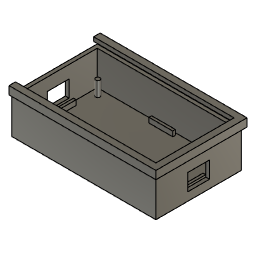
KrabickaSpodek (Autodesk Fusion 360 design; units mm, degrees)
Autodesk Fusion 360 part; units mm, degrees
sketch "Spodek" plane through (0, 0, 0) normal (0, 0, 1) x (1, 0, 0)
  line L0 (0, 0) -> (61, 0)
  line L1 (61, 0) -> (61, 34)
  line L2 (61, 34) -> (0, 34)
  line L3 (0, 34) -> (0, 0)
  line L4 (-1, 35) -> (62, 35)
  line L5 (62, 35) -> (62, -1)
  line L6 (62, -1) -> (-1, -1)
  line L7 (-1, -1) -> (-1, 35)
  line L8 (-2.7, -2.7) -> (-2.7, 36.7) construction
  line L9 (63.7, 36.7) -> (-2.7, 36.7) construction
  line L10 (63.7, -2.7) -> (63.7, 36.7) construction
  line L11 (63.7, -2.7) -> (-2.7, -2.7) construction
  line L12 (-2.7, -2.7) -> (63.7, -2.7)
  line L13 (63.7, -2.7) -> (63.7, 36.7)
  line L14 (63.7, 36.7) -> (-2.7, 36.7)
  line L15 (-2.7, 36.7) -> (-2.7, -2.7)
  dimension "d1" = 61
  dimension "d2" = 34
  dimension "d3" = 63
  dimension "d4" = 36
  dimension "d5" = 1.7
  dimension "d6" = 1.7
  dimension "d7" = 1.7
  dimension "d8" = 1.7
  constraint horizontal L0
  constraint vertical L1
  constraint horizontal L2
  constraint vertical L3
  constraint coincident L0.start L3.end
  constraint horizontal L4
  constraint vertical L5
  constraint horizontal L6
  constraint vertical L7
  constraint vertical L8
  constraint perpendicular L8 L9
  constraint perpendicular L9 L10
  constraint perpendicular L10 L11
  constraint horizontal L12
  constraint vertical L13
  constraint horizontal L14
  constraint vertical L15
  measures "d1" distance of L0.start L0.end
  measures "d2" distance of L0.start L2.end
  measures "d3" distance of L4.start L4.end
  measures "d4" distance of L4.start L6.end
  measures "d5" distance of L7 L8
  measures "d6" distance of L4 L9
  measures "d7" distance of L5 L10
  measures "d8" distance of L6 L11
sketch "TotoNevim" plane through (0, 0, 0) normal (0, 0, 1) x (1, 0, 0)
extrude "Extrude1" add sketch "Spodek" along normal blind 12 contours L12 L13 L14 L15 makes body 1
extrude "Extrude2" add sketch "Spodek" along normal blind 1.5 contours L0 L1 L2 L3 | L4 L5 L6 L7 bodies 1
sketch "Sketch3" plane through (0, 0, 1.5) normal (0, 0, 1) x (-1, 0, 0)
  line L0 (1, 1) -> (-62, 1)
  line L1 (-62, 1) -> (-62, -35)
  line L2 (-62, -35) -> (1, -35)
  line L3 (1, -35) -> (1, 1)
  line L4 (-59.78, -32.78) -> (-1.22, -32.78)
  line L5 (-1.22, -32.78) -> (-1.22, -1.22)
  line L6 (-1.22, -1.22) -> (-59.78, -1.22)
  line L7 (-59.78, -1.22) -> (-59.78, -32.78)
  line L8 (-61, 0) -> (-61, -34)
  line L9 (0, 0) -> (-61, 0)
  line L10 (0, -34) -> (0, 0)
  line L11 (-61, -34) -> (0, -34)
  dimension "d13" = 1.22
  dimension "d14" = 1.22
  dimension "d15" = 1.22
  dimension "d16" = 1.22
  constraint horizontal L4
  constraint vertical L5
  constraint horizontal L6
  constraint vertical L7
  measures "d13" distance of L7 L8
  measures "d14" distance of L6 L9
  measures "d15" distance of L5 L10
  measures "d16" distance of L4 L11
extrude "Extrude3" add sketch "Sketch3" along normal blind 1.8 contours L8 L9 L10 L11 bodies 1
extrude "Extrude4" add 1 faces at (20, -2.1333, 12) along direction (0, 0, 1) blind 5.243 on bodies 1 bodies 1
extrude "Extrude5" add 1 faces at (20, -2.1333, 17.243) along direction (0, 0, 1) blind 0.021 on bodies 1 bodies 1
sketch "Prurez1" plane through (-2.7, 0, 0) normal (-1, 0, 0) x (0, -1, 0)
  line L0 (-36.7, 0) -> (2.7, 0)
  line L1 (2.7, 0) -> (2.7, 17.264)
  line L2 (2.7, 17.264) -> (-36.7, 17.264)
  line L3 (-36.7, 17.264) -> (-36.7, 0)
  line L4 (-12, 3.3) -> (-12, 11) construction
  line L5 (0, 1.5) -> (0, 3.3) construction
  line L6 (-22, 11) -> (-22, 3.3) construction
  line L7 (-34, 3.3) -> (-34, 11) construction
  line L8 (-35, 1.5) -> (-35, 17.264) construction
  line L9 (-22, 11) -> (-12, 11) construction
  line L10 (-12, 11) -> (-12, 3.3) construction
  line L11 (-12, 3.3) -> (-22, 3.3) construction
  line L12 (-22, 3.3) -> (-22, 11) construction
  line L13 (-22, 11) -> (-12, 11)
  line L14 (-12, 11) -> (-12, 3.3)
  line L15 (-12, 3.3) -> (-22, 3.3)
  line L16 (-22, 3.3) -> (-22, 11)
  dimension "d23" = 7.7
  dimension "d24" = 12
  dimension "d25" = 12
  dimension "d26" = 1
  constraint perpendicular L2 L4
  constraint parallel L4 L6
  constraint perpendicular L2 L7
  constraint horizontal L9
  constraint vertical L10
  constraint horizontal L11
  constraint vertical L12
  constraint horizontal L13
  constraint vertical L14
  constraint horizontal L15
  constraint vertical L16
  measures "d23" distance of L4.start L4.end
  measures "d24" distance of L4 L5
  measures "d25" distance of L6 L7
  measures "d26" distance of L7 L8
extrude "Extrude6" cut sketch "Prurez1" against normal up to surface (66.4 mm away) contours L13 L14 L15 L16 bodies 1
sketch "Sketch5" plane through (0, 0, 17.264) normal (0, 0, 1) x (-1, 0, 0)
  line L0 (-62, 1) -> (1, 1)
  line L1 (1, 1) -> (1, -35)
  line L2 (1, -35) -> (-62, -35)
  line L3 (-62, -35) -> (-62, 1)
  line L4 (2.7, -36.7) -> (2.7, 2.7)
  line L5 (2.7, 2.7) -> (-63.7, 2.7)
  line L6 (-63.7, 2.7) -> (-63.7, -36.7)
  line L7 (-63.7, -36.7) -> (2.7, -36.7)
  line L8 (2.7, -36.7) -> (-63.7, -36.7)
  line L9 (-63.7, -36.7) -> (-63.7, 2.7)
  line L10 (-63.7, 2.7) -> (2.7, 2.7)
  line L11 (2.7, 2.7) -> (2.7, -36.7)
  line L12 (1, -35) -> (-62, -35)
  line L13 (-62, -35) -> (-62, 1)
  line L14 (-62, 1) -> (1, 1)
  line L15 (1, 1) -> (1, -35)
  constraint horizontal L8
  constraint vertical L9
  constraint horizontal L10
  constraint vertical L11
  constraint coincident L5.end L6.start
  constraint coincident L4.start L7.end
  constraint horizontal L12
  constraint vertical L13
  constraint horizontal L14
  constraint vertical L15
  constraint coincident L0.start L3.end
  constraint coincident L1.end L2.start
extrude "Extrude7" add sketch "Sketch5" along normal blind 3.7 bodies 1
sketch "Sketch6" plane through (-2.7, 0, 0) normal (-1, 0, 0) x (0, -1, 0)
  line L0 (-22, 3.3) -> (-22, 11)
  line L1 (-22, 11) -> (-12, 11)
  line L2 (-12, 11) -> (-12, 3.3)
  line L3 (-12, 3.3) -> (-22, 3.3)
  line L4 (-36.7, 0) -> (2.7, 0)
  line L5 (2.7, 0) -> (2.7, 20.964)
  line L6 (2.7, 20.964) -> (-36.7, 20.964)
  line L7 (-36.7, 20.964) -> (-36.7, 0)
  line L8 (-35, 17.264) -> (1.0001, 17.264)
  line L9 (1.0001, 17.264) -> (1.0001, 20.964)
  line L10 (1.0001, 20.964) -> (-35, 20.964)
  line L11 (-35, 20.964) -> (-35, 17.264)
  line L12 (-36.7, 17.264) -> (2.7, 17.264)
  constraint horizontal L8
  constraint vertical L9
  constraint horizontal L10
  constraint vertical L11
  constraint coincident L6 L9.end
  constraint coincident L8.start L12
extrude "Extrude8" cut sketch "Sketch6" against normal up to surface (64.7 mm away) contours L6 L8 L9 L10 L11 L12 bodies 1
sketch "BokFront" plane through (0, -2.7, 0) normal (0, -1, 0) x (1, 0, 0)
  line L0 (-2.7, 0) -> (63.7, 0)
  line L1 (63.7, 0) -> (63.7, 20.964)
  line L2 (63.7, 20.964) -> (-2.7, 20.964)
  line L3 (-2.7, 20.964) -> (-2.7, 0)
  line L4 (-2.7, 20.964) -> (63.7, 20.964)
  line L5 (63.7, 20.964) -> (63.7, 17.264)
  line L6 (63.7, 17.264) -> (-2.7, 17.264)
  line L7 (-2.7, 17.264) -> (-2.7, 20.964)
  point P0 (63.7, 17.264)
  constraint horizontal L4
  constraint vertical L5
  constraint horizontal L6
  constraint vertical L7
  constraint coincident P0 L5.end
  constraint coincident L2.end L3.start
sketch "BokRight" plane through (63.7, 0, 0) normal (1, 0, 0) x (0, 1, 0)
  line L0 (22, 11) -> (22, 3.3)
  line L1 (22, 3.3) -> (12, 3.3)
  line L2 (12, 3.3) -> (12, 11)
  line L3 (12, 11) -> (22, 11)
  line L4 (-2.7, 0) -> (36.7, 0)
  line L5 (36.7, 0) -> (36.7, 20.964)
  line L6 (36.7, 20.964) -> (-2.7, 20.964)
  line L7 (-2.7, 20.964) -> (-2.7, 0)
  line L8 (-2.7, 20.964) -> (36.7, 20.964)
  line L9 (36.7, 20.964) -> (36.7, 17.264)
  line L10 (36.7, 17.264) -> (-2.7, 17.264)
  line L11 (-2.7, 17.264) -> (-2.7, 20.964)
  point P0 (36.7, 17.264)
  constraint horizontal L8
  constraint vertical L9
  constraint horizontal L10
  constraint vertical L11
  constraint coincident P0 L9.end
  constraint coincident L6.end L7.start
sketch "BokBack" plane through (0, 36.7, 0) normal (0, 1, 0) x (-1, 0, 0)
  line L0 (-63.7, 0) -> (2.7, 0)
  line L1 (2.7, 0) -> (2.7, 20.964)
  line L2 (2.7, 20.964) -> (-63.7, 20.964)
  line L3 (-63.7, 20.964) -> (-63.7, 0)
  line L4 (-63.7, 20.964) -> (2.7, 20.964)
  line L5 (2.7, 20.964) -> (2.7, 17.264)
  line L6 (2.7, 17.264) -> (-63.7, 17.264)
  line L7 (-63.7, 17.264) -> (-63.7, 20.964)
  point P0 (2.7, 17.264)
  constraint horizontal L4
  constraint vertical L5
  constraint horizontal L6
  constraint vertical L7
  constraint coincident P0 L5.end
  constraint coincident L2.end L3.start
extrude "Extrude9" add sketch "BokBack" along normal blind 1.3 contours L1 L2 L3 L4 L5 L6 L7 bodies 1
extrude "Extrude10" add sketch "BokFront" along normal blind 1.3 contours L1 L2 L3 L4 L5 L6 L7 bodies 1
extrude "Extrude11" add sketch "BokRight" along normal blind 1.3 contours L5 L6 L7 L8 L9 L10 L11 bodies 1
extrude "Extrude12" add 1 faces at (63.7, 37.5667, 19.7307) along direction (1, 0, 0) blind 1.3 on bodies 1 bodies 1
extrude "Extrude13" add 1 faces at (63.7, -3.1333, 19.7307) along direction (1, 0, 0) blind 1.3 on bodies 1 bodies 1
sketch "Sketch10" plane through (-2.7, 0, 0) normal (-1, 0, 0) x (0, -1, 0)
  line L0 (-35, 17.264) -> (-35, 20.964)
  line L1 (-35, 20.964) -> (-38, 20.964)
  line L2 (-38, 20.964) -> (-38, 17.264)
  line L3 (-38, 17.264) -> (-36.7, 17.264)
  line L4 (-36.7, 17.264) -> (-36.7, 0)
  line L5 (-36.7, 0) -> (2.7, 0)
  line L6 (2.7, 0) -> (2.7, 17.264)
  line L7 (2.7, 17.264) -> (4, 17.264)
  line L8 (4, 17.264) -> (4, 20.964)
  line L9 (4, 20.964) -> (1.0001, 20.964)
  line L10 (1.0001, 20.964) -> (1.0001, 17.264)
  line L11 (1.0001, 17.264) -> (-35, 17.264)
  line L12 (-22, 3.3) -> (-22, 11)
  line L13 (-22, 11) -> (-12, 11)
  line L14 (-12, 11) -> (-12, 3.3)
  line L15 (-12, 3.3) -> (-22, 3.3)
  line L16 (4, 17.264) -> (2.7, 16)
  line L17 (-38, 17.264) -> (-36.7, 16)
  constraint coincident L7.end L8.start
  constraint coincident L6 L16.end
  constraint coincident L2.end L3.start
  constraint coincident L4 L17.end
extrude "Extrude14" add sketch "Sketch10" against normal up to surface (67.7 mm away) contours L3 L4 L17 | L6 L7 L16 bodies 1
sketch "Sketch11" plane through (0, -2.7, 0) normal (0, 1, 0) x (-1, 0, 0)
  line L0 (-63.7, 16) -> (-63.7, 17.264)
  line L1 (-63.7, 17.264) -> (-65, 17.264)
  line L2 (-65, 17.264) -> (-65, 16)
  line L3 (-65, 16) -> (-63.7, 16)
  line L4 (-65, 17.264) -> (-63.7, 16)
  constraint coincident L1.end L2.start
  constraint coincident L0.start L3.end
extrude "Extrude15" add sketch "Sketch11" along normal blind 39.4 contours L0 L1 L4 bodies 1
extrude "Extrude16" cut 1 faces at (64.5667, -2.7, 16.4213) along direction (0, -1, 0) blind 5.3 on bodies 1 bodies 1
extrude "Extrude17" cut 1 faces at (64.5667, 36.7, 16.4213) along direction (0, 1, 0) blind 1.9 on bodies 1 bodies 1
sketch "Sketch12" plane through (-2.7, 35.85, 19.114) normal (-1, 0, 0) x (0, -1, 0)
  line L0 (-0.85, 0) -> (0.85, 0)
  line L1 (0.85, 0) -> (0.85, -1.85)
  line L2 (0.85, -1.85) -> (-0.85, -1.85)
  line L3 (-0.85, -1.85) -> (-0.85, 0)
  line L4 (-0.85, 1.85) -> (-0.85, -19.114)
  line L5 (36.8501, -1.85) -> (38.55, -1.85)
  line L6 (38.55, -1.85) -> (38.55, 0)
  line L7 (38.55, 0) -> (36.8501, 0)
  line L8 (36.8501, 0) -> (36.8501, -1.85)
  line L9 (38.55, -19.114) -> (38.55, 1.85)
  point P0 (0.85, -1.85)
  point P1 (36.8501, -1.85)
  constraint horizontal L0
  constraint vertical L1
  constraint horizontal L2
  constraint vertical L3
  constraint coincident P0 L1.end
  constraint coincident L0.start L4
  constraint horizontal L5
  constraint vertical L6
  constraint horizontal L7
  constraint vertical L8
  constraint coincident L6.end L9
  constraint coincident P1 L5.start
extrude "Extrude18" cut sketch "Sketch12" against normal blind 64.7 bodies 1
sketch "Sketch13" plane through (62, 0, 0) normal (-1, 0, 0) x (0, -1, 0)
  line L0 (-35, 17.264) -> (-35, 1.5)
  line L1 (-35, 1.5) -> (1, 1.5)
  line L2 (1, 1.5) -> (1, 17.264)
  line L3 (1.0001, 17.264) -> (2.7, 17.264)
  line L4 (2.7, 17.264) -> (2.7, 19.114)
  line L5 (2.7, 19.114) -> (1.0001, 19.114)
  line L6 (1, 19.114) -> (1, 20.964)
  line L7 (1, 20.964) -> (-35, 20.964)
  line L8 (-35, 20.964) -> (-35, 19.114)
  line L9 (-35, 19.114) -> (-36.7, 19.114)
  line L10 (-36.7, 19.114) -> (-36.7, 17.264)
  line L11 (-36.7, 17.264) -> (-35, 17.264)
  line L12 (-22, 3.3) -> (-22, 11)
  line L13 (-22, 11) -> (-12, 11)
  line L14 (-12, 11) -> (-12, 3.3)
  line L15 (-12, 3.3) -> (-22, 3.3)
  line L16 (-36.7, 19.114) -> (2.7, 19.114)
  line L17 (2.7, 19.114) -> (2.7, 17.264)
  line L18 (2.7, 17.264) -> (-36.7, 17.264)
  line L19 (-36.7, 17.264) -> (-36.7, 19.114)
  constraint horizontal L16
  constraint vertical L17
  constraint horizontal L18
  constraint vertical L19
  constraint coincident L3.end L4.start
  constraint coincident L9.end L10.start
extrude "Extrude19" cut sketch "Sketch13" against normal blind 1.7 contours L3 L4 L5 L9 L10 L11 L16 L17 L18 L19 bodies 1
sketch "Sketch14" plane through (0, 0, 3.3) normal (0, 0, 1) x (-1, 0, 0)
  line L0 (0, -34) -> (0, 0)
  line L1 (0, 0) -> (-61, 0)
  line L2 (-61, 0) -> (-61, -34)
  line L3 (-61, -34) -> (0, -34)
  line L4 (-1.22, -1.22) -> (-1.22, -32.78)
  line L5 (-1.22, -32.78) -> (-59.78, -32.78)
  line L6 (-59.78, -32.78) -> (-59.78, -1.22)
  line L7 (-59.78, -1.22) -> (-1.22, -1.22)
  circle A0 centre (-58.6, -31.85) radius 1
  line L8 (-61, -17) -> (0, -17) construction
  circle A1 centre (-58.6, -2.15) radius 1
  line L9 (-30.5, -34) -> (-30.5, 0) construction
  circle A2 centre (-2.4, -31.85) radius 1
  circle A3 centre (-2.4, -2.15) radius 1
  point P0 (-58.6, -31.85)
  dimension "d55" = 2.15
  dimension "d56" = 2.4
  dimension "d57" = 2
  constraint coincident P0 A0.centre
  constraint midpoint L2 L8.start
  constraint midpoint L0 L8.end
  constraint symmetric A0 L8 A1
  constraint midpoint L3 L9.start
  constraint midpoint L1 L9.end
  constraint symmetric A0 L9 A2
  constraint symmetric A1 L9 A3
  measures "d55" distance of L3 P0
  measures "d56" distance of L2 P0
  measures "d57" diameter of A0
extrude "Extrude20" add sketch "Sketch14" along normal blind 5 separate body contours L7 A3 | L5 A2 | L7 A1 | L5 A0 picked at (-2.6077, -1.9583) picked at (-2.278, -32.1598) picked at (-58.2997, -2.1959) picked at (-58.3551, -31.7867) makes body 2 at (59.2633, 32.5983, 6.6333) makes body 3 at (59.1416, 2.9907, 6.6333) makes body 4 at (3.0633, 32.5983, 6.6333) makes body 5 at (2.8103, 3.062, 6.6333)
extrude "Extrude21" add 4 faces at (2.6077, 1.9583, 3.3) (2.278, 32.1598, 3.3) (58.3551, 31.7867, 3.3) (58.2997, 2.1959, 3.3) along direction (0, 0, -1) blind 2 on bodies 2 3 4 5 bodies 5 1 2 3 4
extrude "Extrude22" add 1 faces at (39.7441, 0.4067, 3.3) along direction (0, 0, 1) blind 0.5 on bodies 5 bodies 5
sketch "Sketch15" plane through (0, 0, 3.8) normal (0, 0, 1) x (-1, 0, 0)
  line L0 (0, -34) -> (0, 0)
  line L1 (0, 0) -> (-61, 0)
  line L2 (-61, 0) -> (-61, -34)
  line L3 (-61, -34) -> (0, -34)
  line L4 (-1.22, -1.22) -> (-1.22, -32.78)
  line L5 (-1.22, -32.78) -> (-2.0324, -32.78)
  line L6 (-2.0324, -32.78) -> (-2.7676, -32.78)
  line L7 (-2.7676, -32.78) -> (-58.2324, -32.78)
  line L8 (-58.2324, -32.78) -> (-58.9676, -32.78)
  line L9 (-58.9676, -32.78) -> (-59.78, -32.78)
  line L10 (-59.78, -32.78) -> (-59.78, -1.22)
  line L11 (-59.78, -1.22) -> (-58.9676, -1.22)
  line L12 (-58.9676, -1.22) -> (-58.2324, -1.22)
  line L13 (-58.2324, -1.22) -> (-2.7676, -1.22)
  line L14 (-2.7676, -1.22) -> (-2.0324, -1.22)
  line L15 (-2.0324, -1.22) -> (-1.22, -1.22)
  line L16 (0, -34) -> (-1.22, -34)
  line L17 (-1.22, -34) -> (-1.22, -23)
  line L18 (-1.22, -23) -> (0, -23)
  line L19 (0, -23) -> (0, -34)
  line L20 (0, 0) -> (-1.22, 0)
  line L21 (-1.22, 0) -> (-1.22, -11)
  line L22 (-1.22, -11) -> (0, -11)
  line L23 (0, -11) -> (0, 0)
  line L24 (0, 0) -> (-25, 0)
  line L25 (-25, 0) -> (-25, -1.22)
  line L26 (-25, -1.22) -> (0, -1.22)
  line L27 (0, -1.22) -> (0, 0)
  line L28 (-61, 0) -> (-36, 0)
  line L29 (-36, 0) -> (-36, -1.22)
  line L30 (-36, -1.22) -> (-61, -1.22)
  line L31 (-61, -1.22) -> (-61, 0)
  line L32 (-61, 0) -> (-59.78, 0)
  line L33 (-59.78, 0) -> (-59.78, -11)
  line L34 (-59.78, -11) -> (-61, -11)
  line L35 (-61, -11) -> (-61, 0)
  line L36 (-61, -34) -> (-59.78, -34)
  line L37 (-59.78, -34) -> (-59.78, -23)
  line L38 (-59.78, -23) -> (-61, -23)
  line L39 (-61, -23) -> (-61, -34)
  line L40 (0, -34) -> (-25, -34)
  line L41 (-25, -34) -> (-25, -32.78)
  line L42 (-25, -32.78) -> (0, -32.78)
  line L43 (0, -32.78) -> (0, -34)
  line L44 (-61, -34) -> (-36, -34)
  line L45 (-36, -34) -> (-36, -32.78)
  line L46 (-36, -32.78) -> (-61, -32.78)
  line L47 (-61, -32.78) -> (-61, -34)
  dimension "d64" = 11
  dimension "d65" = 11
  dimension "d66" = 25
  dimension "d67" = 25
  dimension "d68" = 11
  dimension "d69" = 11
  dimension "d70" = 25
  dimension "d71" = 25
  constraint horizontal L16
  constraint vertical L17
  constraint horizontal L18
  constraint vertical L19
  constraint coincident L0.start L3.end
  constraint horizontal L20
  constraint vertical L21
  constraint horizontal L22
  constraint vertical L23
  constraint coincident L0.end L1.start
  constraint horizontal L24
  constraint vertical L25
  constraint horizontal L26
  constraint vertical L27
  constraint horizontal L28
  constraint vertical L29
  constraint horizontal L30
  constraint vertical L31
  constraint coincident L1.end L2.start
  constraint horizontal L32
  constraint vertical L33
  constraint horizontal L34
  constraint vertical L35
  constraint horizontal L36
  constraint vertical L37
  constraint horizontal L38
  constraint vertical L39
  constraint coincident L2.end L3.start
  constraint horizontal L40
  constraint vertical L41
  constraint horizontal L42
  constraint vertical L43
  constraint horizontal L44
  constraint vertical L45
  constraint horizontal L46
  constraint vertical L47
  measures "d64" distance of L0.start L18.end
  measures "d65" distance of L0.end L22.end
  measures "d66" distance of L0.end L24.end
  measures "d67" distance of L1.end L28.end
  measures "d68" distance of L1.end L34.end
  measures "d69" distance of L2.end L38.end
  measures "d70" distance of L0.start L40.end
  measures "d71" distance of L2.end L44.end
extrude "Extrude23" cut sketch "Sketch15" against normal blind 2.3 contours L0 L3 L16 L17 L19 L40 L42 L43 | L3 L5 L6 L7 L17 L40 L41 L42 bodies 5
extrude "Extrude24" cut sketch "Sketch15" against normal blind 2.3 contours L3 L7 L8 L9 L37 L44 L45 L46 | L2 L3 L36 L37 L39 L44 L46 L47 bodies 5
extrude "Extrude25" cut sketch "Sketch15" against normal blind 2.3 contours L2 L10 L37 L38 L39 L46 bodies 5
extrude "Extrude26" cut sketch "Sketch15" against normal blind 2.3 contours L0 L4 L21 L22 L23 L26 | L0 L1 L20 L21 L23 L24 L26 L27 | L1 L13 L14 L15 L21 L24 L25 L26 | L2 L10 L30 L33 L34 L35 | L1 L11 L12 L13 L28 L29 L30 L33 | L1 L2 L28 L30 L31 L32 L33 L35 bodies 5
extrude "Extrude27" cut sketch "Sketch15" against normal blind 2.3 contours L0 L4 L17 L18 L19 L42 bodies 5
extrude "Extrude28" cut 1 faces at (63.1333, 18.6667, 11) along direction (0, 0, 1) blind 0.5 on bodies 5 bodies 5
extrude "Extrude29" cut 1 faces at (-2.1333, 18.6667, 11) along direction (0, 0, 1) blind 0.5 on bodies 5 bodies 5
extrude "Extrude30" add 1 faces at (-2.1333, 15.3333, 3.3) along direction (0, 0, 1) blind 0.5 on bodies 5 bodies 5
extrude "Extrude31" add 1 faces at (63.1333, 15.3333, 3.3) along direction (0, 0, 1) blind 0.5 on bodies 5 bodies 5
extrude "Extrude32" add 1 faces at (63.7, 10.4333, 17.8807) along direction (-1, 0, 0) blind 1.7 on bodies 5 bodies 5
equation "d19 = 14 mm - 8.757 mm"
equation "d21 = 14 mm - 13.979 mm"
equation "d33 = 3 mm - 1.70 mm"
equation "d35 = 3 mm - 1.70 mm"
equation "d37 = 3 mm - 1.70 mm"
